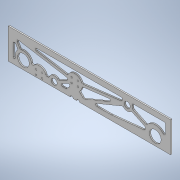
# Autodesk Inventor part: Left right side
Saved by Autodesk Inventor 2021 (Build 250183000, 183)
## iProperties
Created: 2020-09-10
Part Number: Left right side
Material: Generic
Document SubType Name: Modeling
Designer: deli
Density: 1 g/cm^3
Appearance: Default
Author: deli
Autodesk Inventor part; units mm, degrees
ref_plane "YZ Plane" through (0, 0, 0) normal (1, 0, 0) x (0, 1, 0)
ref_plane "XZ Plane" through (0, 0, 0) normal (0, 1, 0) x (-1, 0, 0)
ref_plane "XY Plane" through (0, 0, 0) normal (0, 0, 1) x (1, 0, 0)
sketch "Sketch2" plane through (0, 0, 0) normal (0, 0, 1) x (1, 0, 0)
  arc A0 (94.3199, 17.2212) -> (64.105, 23.0545) centre (77.47, 11.1125) ccw
  arc A1 (58.6141, 24.5997) -> (64.105, 23.0545) centre (61.7375, 25.17) ccw
  arc A2 (58.6141, 24.5997) -> (32.5433, 40.9528) centre (38.1, 20.8534) ccw
  arc A3 (28.9694, 42.3884) -> (32.5433, 40.9528) centre (31.6972, 44.013) ccw
  line L0 (22.4136, 53.3956) -> (28.9694, 42.3884)
  arc A4 (25.6563, 58.1532) -> (22.4136, 53.3956) centre (25.1414, 55.0203) ccw
  line L1 (146.0424, 38.3696) -> (25.6563, 58.1532)
  arc A5 (148.6731, 35.6676) -> (146.0424, 38.3696) centre (145.5275, 35.2367) ccw
  arc A6 (148.6731, 35.6676) -> (148.7334, 35.2616) centre (166.8823, 38.1625) ccw
  arc A7 (147.0007, 31.9121) -> (148.7334, 35.2616) centre (145.5982, 34.7605) ccw
  line L2 (127.4522, 22.2866) -> (147.0007, 31.9121)
  arc A8 (123.959, 22.7455) -> (127.4522, 22.2866) centre (126.0497, 25.1351) ccw
  arc A9 (123.959, 22.7455) -> (102.6424, 17.3068) centre (115.1699, 12.7) ccw
  arc A10 (99.7961, 15.2304) -> (102.6424, 17.3068) centre (99.6625, 18.4026) ccw
  line L3 (97.4383, 15.1312) -> (99.7961, 15.2304)
  arc A11 (94.3199, 17.2212) -> (97.4383, 15.1312) centre (97.3048, 18.3033) ccw
  line L4 (282.9805, 63.5) -> (71.1793, 63.5)
  arc A12 (285.9117, 59.1048) -> (282.9805, 63.5) centre (282.9805, 60.325) ccw
  arc A13 (285.9117, 59.1048) -> (285.3869, 57.5952) centre (298.2343, 53.975) ccw
  arc A14 (282.7104, 55.3041) -> (285.3869, 57.5952) centre (282.3309, 58.4564) ccw
  line L5 (186.9529, 43.7766) -> (282.7104, 55.3041)
  arc A15 (183.6728, 45.6375) -> (186.9529, 43.7766) centre (186.5734, 46.9288) ccw
  arc A16 (183.6728, 45.6375) -> (150.4292, 46.3536) centre (166.8823, 38.1625) ccw
  arc A17 (147.0721, 44.6356) -> (150.4292, 46.3536) centre (147.5869, 47.7686) ccw
  line L6 (70.6644, 57.192) -> (147.0721, 44.6356)
  arc A18 (71.1793, 63.5) -> (70.6644, 57.192) centre (71.1793, 60.325) ccw
  arc A19 (23.0737, 35.3128) -> (17.6991, 16.5328) centre (38.1, 20.8534) ccw
  arc A20 (14.593, 12.7) -> (17.6991, 16.5328) centre (14.593, 15.875) ccw
  arc A21 (12.7, 15.6047) -> (14.593, 12.7) centre (15.875, 15.6047) ccw
  line L7 (12.7, 45.7598) -> (12.7, 15.6047)
  arc A22 (18.6028, 47.3844) -> (12.7, 45.7598) centre (15.875, 45.7598) ccw
  line L8 (23.5138, 39.139) -> (18.6028, 47.3844)
  arc A23 (23.0737, 35.3128) -> (23.5138, 39.139) centre (20.7859, 37.5143) ccw
  arc A24 (186.8127, 14.2677) -> (180.4773, 20.3952) centre (166.8823, 0) ccw
  arc A25 (179.9764, 25.2651) -> (180.4773, 20.3952) centre (182.2383, 23.037) ccw
  arc A26 (179.9764, 25.2651) -> (184.9672, 34.8859) centre (166.8823, 38.1625) ccw
  arc A27 (187.7118, 37.4721) -> (184.9672, 34.8859) centre (188.0913, 34.3199) ccw
  line L9 (252.2114, 45.2367) -> (187.7118, 37.4721)
  arc A28 (253.7976, 39.1478) -> (252.2114, 45.2367) centre (252.5909, 42.0845) ccw
  line L10 (190.6011, 13.1791) -> (253.7976, 39.1478)
  arc A29 (186.8127, 14.2677) -> (190.6011, 13.1791) centre (189.3944, 16.1158) ccw
  line L11 (287.4494, 46.1107) -> (221.0154, 18.8117)
  arc A30 (287.4494, 46.1107) -> (308.5983, 45.5638) centre (298.2343, 53.975) ccw
  line L12 (341.7551, 29.8899) -> (308.5983, 45.5638)
  arc A31 (343.4984, 26.3343) -> (341.7551, 29.8899) centre (340.3982, 27.0194) ccw
  arc A32 (343.4984, 26.3343) -> (343.0855, 23.9175) centre (368.3, 20.8534) ccw
  arc A33 (340.2606, 21.1424) -> (343.0855, 23.9175) centre (339.9337, 24.3005) ccw
  line L13 (258.881, 12.7169) -> (340.2606, 21.1424)
  arc A34 (258.554, 12.7) -> (258.881, 12.7169) centre (258.554, 15.875) ccw
  line L14 (222.2222, 12.7) -> (258.554, 12.7)
  arc A35 (221.0154, 18.8117) -> (222.2222, 12.7) centre (222.2222, 15.875) ccw
  arc A36 (134.5804, 18.7185) -> (135.9845, 12.695) centre (135.9829, 15.87) ccw
  line L15 (149.8057, 26.2152) -> (134.5804, 18.7185)
  arc A37 (153.5171, 25.5462) -> (149.8057, 26.2152) centre (151.2083, 23.3668) ccw
  arc A38 (153.5171, 25.5462) -> (153.7882, 25.2651) centre (166.8823, 38.1625) ccw
  arc A39 (153.2873, 20.3952) -> (153.7882, 25.2651) centre (151.5262, 23.037) ccw
  arc A40 (153.2873, 20.3952) -> (146.8004, 14.0537) centre (166.8823, 0) ccw
  arc A41 (144.2007, 12.6991) -> (146.8004, 14.0537) centre (144.1991, 15.8741) ccw
  line L16 (135.9845, 12.695) -> (144.2007, 12.6991)
  arc A42 (311.5671, 53.3463) -> (310.5568, 59.1048) centre (298.2343, 53.975) ccw
  arc A43 (313.488, 63.5) -> (310.5568, 59.1048) centre (313.488, 60.325) ccw
  line L17 (390.525, 63.5) -> (313.488, 63.5)
  arc A44 (393.7, 60.325) -> (390.525, 63.5) centre (390.525, 60.325) ccw
  line L18 (393.7, 38.8139) -> (393.7, 60.325)
  arc A45 (388.0556, 36.8183) -> (393.7, 38.8139) centre (390.525, 38.8139) ccw
  arc A46 (388.0556, 36.8183) -> (348.323, 36.5403) centre (368.3, 20.8534) ccw
  arc A47 (344.4689, 35.6307) -> (348.323, 36.5403) centre (345.8259, 38.5012) ccw
  line L19 (313.3817, 50.3264) -> (344.4689, 35.6307)
  arc A48 (311.5671, 53.3463) -> (313.3817, 50.3264) centre (314.7386, 53.1968) ccw
  arc A49 (162.6902, 0) -> (155.0743, 0) centre (158.8823, -0.125) ccw
  line L20 (162.6902, 0) -> (171.0743, 0)
  arc A50 (178.6902, 0) -> (171.0743, 0) centre (174.8823, -0.125) ccw
  line L21 (178.6902, 0) -> (406.4, 0)
  line L22 (406.4, 0) -> (406.4, 76.2)
  line L23 (0, 76.2) -> (406.4, 76.2)
  line L24 (0, 0) -> (0, 76.2)
  line L25 (0, 0) -> (155.0743, 0)
  circle A51 centre (69.85, 5.08) radius 1.8542
  circle A52 centre (174.8823, 31.875) radius 1.8542
  circle A53 centre (174.8823, 44.45) radius 1.8542
  circle A54 centre (85.09, 5.08) radius 1.8542
  circle A55 centre (69.85, 17.145) radius 1.8542
  circle A56 centre (158.8823, 31.875) radius 1.8542
  circle A57 centre (158.8823, 44.45) radius 1.8542
  circle A58 centre (85.09, 17.145) radius 1.8542
  circle A59 centre (298.2343, 53.975) radius 7.2517
  circle A60 centre (115.1699, 12.7) radius 7.2517
  circle A61 centre (38.1, 20.8534) radius 14.5034
  circle A62 centre (368.3, 20.8534) radius 14.5034
  point P0 (0, 30.4367)
  dimension "d3" = 14.5034
  dimension "d4" = 14.5034
  constraints: 102 point on circle, 63 centre point, 52 end point, 7 horizontal, 4 vertical, 218 other
  measures "d3" diameter of A60
  measures "d4" diameter of A59
extrude "Extrusion1" add sketch "Sketch2" along normal blind 3.175
equation "\"d4\" = d3"
body "Solid1"
